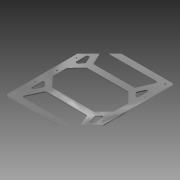
# Autodesk Inventor part: ZBedPlate
Saved by Autodesk Inventor 2015 SP1 (Build 190203100, 203)
## iProperties
Category: Sheet Metal
Created: 2015-01-11
Part Number: ZBedPlate
Material: Steel, Alloy
Document SubType Name: Modeling
Designer: Jack
Density: 7.73 g/cm^3
Appearance: Semi-Polished
Mass: 734.813 g
Surface Area: 727.52 cm^2
Volume: 95.0599 cm^3
Catalog Web Link: N/A
Author: Jack
Title: Bed Support Plate
Autodesk Inventor part; units mm, degrees
ref_plane "YZ Plane" through (0, 0, 0) normal (1, 0, 0) x (0, 1, 0)
ref_plane "XZ Plane" through (0, 0, 0) normal (0, 1, 0) x (-1, 0, 0)
ref_plane "XY Plane" through (0, 0, 0) normal (0, 0, 1) x (1, 0, 0)
sketch "Sketch1" plane through (0, 0, 0) normal (0, 0, 1) x (1, 0, 0)
  line L0 (0, 0) -> (236.5, 0)
  line L1 (236.5, 0) -> (236.5, 296)
  line L2 (236.5, 296) -> (0, 296)
  line L3 (0, 296) -> (0, 0)
  dimension "d0" = 236.5
  dimension "d1" = 296
  constraints: 8 end point, 2 parallel, 1 horizontal, 1 perpendicular
  measures "d0" distance of L0.start L0.end
  measures "d1" distance of L2.end L0.start
extrude "Extrusion1" add sketch "Sketch1" along normal blind 3
sketch "Sketch2" plane through (0, 0, 3) normal (0, 0, 1) x (1, 0, 0)
  line L0 (0, 0) -> (236.5, 0) projected
  line L1 (236.5, 0) -> (236.5, 296) projected
  line L2 (236.5, 296) -> (0, 296) projected
  line L3 (0, 296) -> (0, 0) projected
  line L4 (207.918, 276) -> (27.918, 276)
  line L5 (27.918, 276) -> (52.6323, 223)
  line L6 (52.6323, 223) -> (184.8589, 223)
  line L7 (184.8589, 223) -> (207.918, 276)
  line L8 (216.5, 255.6203) -> (197.8143, 212.6721)
  line L9 (197.8143, 212.6721) -> (216.5, 193.9864)
  line L10 (216.5, 171.3589) -> (184.8589, 203)
  line L11 (216.5, 255.6203) -> (216.5, 193.9864)
  line L12 (184.8589, 203) -> (52.6323, 203)
  line L13 (52.6323, 203) -> (22.4102, 170.0009)
  line L14 (20, 255.1209) -> (39.7942, 212.6721)
  line L15 (39.7942, 212.6721) -> (20, 191.059)
  line L16 (20, 191.059) -> (20, 255.1209)
  line L17 (22.4102, 125.9991) -> (52.6323, 93)
  line L18 (52.6323, 93) -> (184.8589, 93)
  line L19 (184.8589, 93) -> (216.5, 124.6411)
  line L20 (216.5, 124.6411) -> (216.5, 171.3589)
  line L21 (216.5, 102.0136) -> (197.8143, 83.3279)
  line L22 (197.8143, 83.3279) -> (216.5, 40.3797)
  line L23 (216.5, 40.3797) -> (216.5, 102.0136)
  line L24 (20, 104.941) -> (39.7942, 83.3279)
  line L25 (39.7942, 83.3279) -> (20, 40.8791)
  line L26 (20, 40.8791) -> (20, 104.941)
  line L27 (27.918, 20) -> (207.918, 20)
  line L28 (207.918, 20) -> (184.8589, 73)
  line L29 (184.8589, 73) -> (52.6323, 73)
  line L30 (52.6323, 73) -> (27.918, 20)
  line L31 (22.4102, 125.9991) -> (22.4102, 170.0009)
  dimension "d19" = 65
  dimension "d29" = 110
  dimension "d31" = 20
  dimension "d32" = 20
  dimension "d33" = 20
  dimension "d34" = 20
  dimension "d35" = 20
  dimension "d40" = 16
  dimension "d41" = 16
  dimension "d52" = 180
  dimension "d55" = 135
  dimension "d59" = 20
  dimension "d60" = 16
  dimension "d61" = 16
  dimension "d62" = 16
  dimension "d63" = 16
  dimension "d64" = 20
  constraints: 56 end point, 11 parallel, 9 vertical alignment, 8 equal length, 5 vertical, 4 horizontal, 2 horizontal alignment
  measures "d19" angle of L27 L30
  measures "d29" distance between parallel lines of L18 L12
  measures "d31" distance between parallel lines of L6 L12
  measures "d32" distance between parallel lines of L2 L4
  measures "d33" distance between parallel lines of L0 L27
  measures "d34" distance between parallel lines of L1 L11
  measures "d35" distance between parallel lines of L3 L16
  measures "d40" distance between parallel lines of L13 L15
  measures "d41" distance between parallel lines of L9 L10
  measures "d52" distance of L27.start L27.end
  measures "d55" angle of L12 L10
  measures "d59" distance between parallel lines of L29 L18
  measures "d60" distance between parallel lines of L30 L25
  measures "d61" distance between parallel lines of L22 L28
  measures "d62" distance between parallel lines of L8 L7
  measures "d63" distance between parallel lines of L14 L5
  measures "d64" distance between parallel lines of L1 L20
extrude "Extrusion2" cut sketch "Sketch2" against normal up to next contours L7 L6 L5 L4 | L11 L9 L8 | L20 L19 L18 L17 L31 L13 L12 L10 | L14 L15 L16 | L23 L22 L21 | L24 L25 L26 | L30 L29 L28 L27
sketch "Sketch3" plane through (0, 0, 3) normal (0, 0, 1) x (1, 0, 0)
  line L0 (0, 0) -> (236.5, 0) projected
  line L1 (236.5, 0) -> (236.5, 296) projected
  line L2 (236.5, 296) -> (0, 296) projected
  line L3 (0, 296) -> (0, 0) projected
  circle A0 centre (222.5, 282) radius 2.25
  circle A1 centre (14, 148) radius 2.25
  circle A2 centre (222.5, 14) radius 2.25
  dimension "d44" = 4.5
  dimension "d45" = 14
  dimension "d46" = 14
  dimension "d47" = 14
  dimension "d56" = 148
  dimension "d57" = 14
  constraints: 3 centre point, 2 equal radius, 1 vertical alignment
  measures "d44" diameter of A0
  measures "d45" distance from line of L1 A0.centre
  measures "d46" distance from line of L2 A0.centre
  measures "d47" distance from line of L0 A2.centre
  measures "d56" distance from line of L2 A1.centre
  measures "d57" distance from line of L3 A1.centre
extrude "Extrusion3" cut sketch "Sketch3" against normal up to next contours A0 | A1 | A2
fillet "Fillet1" radius 4.7625 28 edges at (27.918, 20, 1.5) (207.918, 20, 1.5) (184.8589, 73, 1.5) (52.6323, 73, 1.5) (20, 40.8791, 1.5) (39.7942, 83.3279, 1.5) (20, 104.941, 1.5) (39.7942, 212.6721, 1.5) (20, 191.059, 1.5) (20, 255.1209, 1.5) (27.918, 276, 1.5) (52.6323, 223, 1.5) (184.8589, 223, 1.5) (207.918, 276, 1.5) (197.8143, 83.3279, 1.5) (216.5, 40.3797, 1.5) (216.5, 102.0136, 1.5) (216.5, 193.9864, 1.5) (197.8143, 212.6721, 1.5) (216.5, 255.6203, 1.5) (216.5, 124.6411, 1.5) (216.5, 171.3589, 1.5) (184.8589, 93, 1.5) (184.8589, 203, 1.5) (52.6323, 203, 1.5) (22.4102, 170.0009, 1.5) (22.4102, 125.9991, 1.5) (52.6323, 93, 1.5)
fillet "Fillet2" radius 5 4 edges at (236.5, 0, 1.5) (0, 0, 1.5) (0, 296, 1.5) (236.5, 296, 1.5)
sketch "Sketch4" plane through (0, 0, 0) normal (0, 0, -1) x (-1, 0, 0)
  line L0 (-182.8862, 203) -> (-54.7286, 203) projected
  line L1 (-54.7286, 93) -> (-182.8862, 93) projected
  line L2 (-236.5, 5) -> (-236.5, 291) projected
  line L3 (0, 291) -> (0, 5) projected
  point P0 (0, 0)
  point P1 (-10, 213)
  point P2 (-226.5, 213)
  point P3 (-10, 83)
  point P4 (-226.5, 83)
  dimension "d65" = 10
  dimension "d66" = 10
  dimension "d67" = 10
  dimension "d68" = 10
  constraints: 2 horizontal alignment, 2 vertical alignment
  measures "d65" distance from line of point (-10, 213) L0
  measures "d66" distance from line of point (-10, 83) L1
  measures "d67" distance from line of L2 point (-226.5, 83)
  measures "d68" distance from line of L3 point (-10, 83)
hole "Hole1" at (10, 213, 0) at (226.5, 213, 0) at (10, 83, 0) at (226.5, 83, 0) direction (0, 0, 1) diameter 4 end through all countersink diameter 8 countersink angle 90
body "Solid1"
